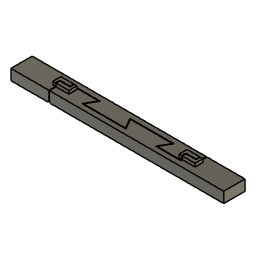
Split Turnout 600mm 15deg (Autodesk Fusion 360 archive; units mm, degrees)
design "Track Joint Parametric"
Autodesk Fusion 360 part; units mm, degrees
sketch "Sketch1" plane through (0, 0, 0) normal (0, 0, 1) x (1, 0, 0)
  line L0 (-20, 2) -> (20, 2)
  line L1 (20, 2) -> (20, -2)
  line L2 (20, -2) -> (-20, -2)
  line L3 (-20, -2) -> (-20, 2)
  line L4 (0, -2) -> (0, 2) construction
  line L5 (-20, 0) -> (20, 0) construction
  line L6 (-11.85, 2) -> (-11.85, -2) construction
  line L7 (11.85, 2) -> (11.85, -2) construction
  line L8 (-12.75, 2) -> (-12.75, -2)
  line L9 (-12.45, 2) -> (-12.45, -2) construction
  line L10 (-11.25, 2) -> (-11.25, -2) construction
  line L11 (-10.95, 2) -> (-10.95, -2)
  line L12 (11.25, 2) -> (11.25, -2) construction
  line L13 (12.45, 2) -> (12.45, -2) construction
  line L14 (10.95, 2) -> (10.95, -2)
  line L15 (12.75, 2) -> (12.75, -2)
  line L16 (-13.35, 0.75) -> (-10.35, 0.75)
  line L17 (-10.35, 0.75) -> (-10.35, -0.75)
  line L18 (-10.35, -0.75) -> (-13.35, -0.75)
  line L19 (-13.35, -0.75) -> (-13.35, 0.75)
  line L20 (10.35, 0.75) -> (13.35, 0.75)
  line L21 (13.35, 0.75) -> (13.35, -0.75)
  line L22 (13.35, -0.75) -> (10.35, -0.75)
  line L23 (10.35, -0.75) -> (10.35, 0.75)
  line L24 (-11.85, 1) -> (-6.3453, 1) construction
  line L25 (-6.3453, 1) -> (-7.5, -1) construction
  line L26 (-7.5, -1) -> (0.5774, -1) construction
  line L27 (0.5774, -1) -> (-0.5774, 1) construction
  line L28 (-0.5774, 1) -> (7.5, 1) construction
  line L29 (7.5, 1) -> (6.3453, -1) construction
  line L30 (6.3453, -1) -> (11.85, -1) construction
  line L31 (-3.4613, -1) -> (-3.4613, 2) construction
  line L32 (3.4613, 1) -> (3.4613, -2) construction
  line L33 (-12.85, 0.05) -> (-10.95, 0.05)
  line L34 (-10.95, 1.05) -> (-6.2587, 1.05)
  line L35 (-6.2587, 1.05) -> (-7.4134, -0.95)
  line L36 (-7.4134, -0.95) -> (0.4907, -0.95)
  line L37 (0.4907, -0.95) -> (-0.664, 1.05)
  line L38 (-0.664, 1.05) -> (7.5866, 1.05)
  line L39 (7.5866, 1.05) -> (6.4319, -0.95)
  line L40 (6.4319, -0.95) -> (10.85, -0.95)
  line L41 (-12.85, 0.05) -> (-12.85, -2)
  line L42 (-12.75, -0.05) -> (-10.85, -0.05)
  line L43 (-10.85, -0.05) -> (-10.85, 0.95)
  line L44 (-10.85, 0.95) -> (-6.4319, 0.95)
  line L45 (-6.4319, 0.95) -> (-7.5866, -1.05)
  line L46 (-7.5866, -1.05) -> (0.664, -1.05)
  line L47 (0.664, -1.05) -> (-0.4907, 0.95)
  line L48 (-0.4907, 0.95) -> (7.4134, 0.95)
  line L49 (7.4134, 0.95) -> (6.2587, -1.05)
  line L50 (6.2587, -1.05) -> (10.95, -1.05)
  line L51 (10.85, -0.95) -> (10.85, -0.903)
  line L52 (10.85, -0.903) -> (10.85, 0.05)
  line L53 (10.85, 0.05) -> (12.75, 0.05)
  line L54 (10.95, -0.05) -> (12.85, -0.05)
  line L55 (12.85, -0.05) -> (12.85, 2)
  line L56 (-12.25, 2) -> (-12.25, -2) construction
  line L57 (-11.45, -2) -> (-11.45, 2) construction
  line L58 (11.45, 2) -> (11.45, -2) construction
  line L59 (12.25, 2) -> (12.25, -2) construction
  point P0 (-6.9226, 0)
  point P1 (6.9226, 0)
  point P2 (-11.85, 0)
  point P3 (11.85, 0)
  dimension "d123" = 40
  dimension "d124" = 1.2
  dimension "d125" = 1.8
  dimension "d127" = 4
  dimension "d128" = 3
  dimension "d129" = 1.5
  dimension "d130" = 30
  dimension "d131" = 2
  dimension "d132" = 15
  dimension "d133" = 0.1
  dimension "d134" = 0.1
  dimension "d136" = 0.1
  dimension "d137" = 0.1
  dimension "d138" = 0.1
  dimension "d139" = 0.1
  dimension "d140" = 0.1
  dimension "d141" = 0.1
  dimension "d142" = 0.1
  dimension "d143" = 0.1
  dimension "d144" = 0.1
  dimension "d145" = 0.1
  dimension "d146" = 0.1
  dimension "d147" = 0.8
  dimension "d161" = 22.5
  constraint horizontal L0
  constraint vertical L1
  constraint horizontal L2
  constraint vertical L3
  constraint coincident L2 L4.start
  constraint coincident L0 L4.end
  constraint coincident L3 L5.start
  constraint coincident L1 L5.end
  constraint perpendicular L0 L4
  constraint perpendicular L1 L5
  constraint symmetric L1 L3 L4
  constraint symmetric L0 L2 L5
  constraint coincident origin L4
  constraint coincident origin L5
  constraint coincident L0 L6.start
  constraint coincident L2 L6.end
  constraint perpendicular L2 L6
  constraint coincident L0 L7.start
  constraint coincident L2 L7.end
  constraint perpendicular L2 L7
  constraint symmetric L4 L6 L7
  constraint coincident L0 L8.start
  constraint coincident L2 L8.end
  constraint perpendicular L2 L8
  constraint coincident L0 L9.start
  constraint coincident L2 L9.end
  constraint perpendicular L2 L9
  constraint coincident L0 L10.start
  constraint coincident L2 L10.end
  constraint perpendicular L2 L10
  constraint coincident L0 L11.start
  constraint coincident L2 L11.end
  constraint perpendicular L2 L11
  constraint symmetric L6 L9 L10
  constraint symmetric L6 L8 L11
  constraint coincident L0 L12.start
  constraint coincident L2 L12.end
  constraint perpendicular L2 L12
  constraint coincident L0 L13.start
  constraint coincident L2 L13.end
  constraint perpendicular L2 L13
  constraint coincident L0 L14.start
  constraint coincident L2 L14.end
  constraint perpendicular L2 L14
  constraint coincident L0 L15.start
  constraint coincident L2 L15.end
  constraint perpendicular L2 L15
  constraint symmetric L7 L14 L15
  constraint symmetric L7 L12 L13
  constraint symmetric L4 L11 L14
  constraint symmetric L4 L10 L12
  constraint horizontal L16
  constraint vertical L17
  constraint horizontal L18
  constraint vertical L19
  constraint symmetric L5 L16 L18
  constraint symmetric L6 L17 L19
  constraint horizontal L20
  constraint vertical L21
  constraint horizontal L22
  constraint vertical L23
  constraint symmetric L5 L20 L22
  constraint symmetric L7 L21 L23
  constraint symmetric L4 L17 L23
  constraint collinear L18 L22
  constraint coincident L6 L24.start
  constraint coincident L7 L30.end
  constraint parallel L5 L30
  constraint parallel L5 L28
  constraint parallel L5 L26
  constraint parallel L5 L24
  constraint coincident origin L27
  constraint collinear L26 L30
  constraint coincident L25 P0
  constraint coincident L29 P1
  constraint coincident L5 P1
  constraint coincident L5 P0
  constraint symmetric L4 P0 P1
  constraint coincident L26 L31.start
  constraint coincident L0 L31.end
  constraint perpendicular L0 L31
  constraint symmetric L25 L27 L31
  constraint coincident L28 L32.start
  constraint coincident L2 L32.end
  constraint perpendicular L2 L32
  constraint symmetric L27 L29 L32
  constraint coincident L11 L33.end
  constraint perpendicular L11 L33
  constraint coincident L11 L34.start
  constraint parallel L30 L40
  constraint parallel L29 L39
  constraint parallel L28 L38
  constraint parallel L27 L37
  constraint parallel L26 L36
  constraint parallel L25 L35
  constraint parallel L24 L34
  constraint coincident L2 L41.end
  constraint parallel L8 L41
  constraint coincident L8 L42.start
  constraint parallel L26 L46
  constraint parallel L25 L45
  constraint parallel L24 L44
  constraint parallel L11 L43
  constraint parallel L33 L42
  constraint parallel L28 L48
  constraint parallel L29 L49
  constraint parallel L30 L50
  constraint parallel L27 L47
  constraint coincident L14 L50.end
  constraint perpendicular L40 L51
  constraint coincident L15 L53.end
  constraint coincident L14 L54.start
  constraint coincident L0 L55.end
  constraint parallel L15 L55
  constraint parallel L5 L54
  constraint parallel L53 L54
  constraint parallel L14 L52
  constraint coincident L0 L56.start
  constraint perpendicular L0 L56
  constraint coincident L2 L56.end
  constraint coincident L2 L57.start
  constraint coincident L0 L57.end
  constraint perpendicular L0 L57
  constraint symmetric L6 L56 L57
  constraint coincident L0 L58.start
  constraint coincident L2 L58.end
  constraint perpendicular L2 L58
  constraint coincident L0 L59.start
  constraint coincident L2 L59.end
  constraint perpendicular L2 L59
  constraint symmetric L7 L58 L59
  constraint symmetric L4 L57 L58
  constraint coincident L6 P2
  constraint coincident L5 P2
  constraint coincident L7 P3
  constraint coincident L5 P3
  measures "d123" distance of L1 L3
  measures "d124" distance of L9 L10
  measures "d125" distance of L8 L11
  measures "d127" distance of L0 L2
  measures "d128" distance of L17 L19
  measures "d129" distance of L16 L18
  measures "d130" angle of L4 L27
  measures "d131" distance of L28 L30
  measures "d132" horizontal distance of L25.end L28.end
  measures "d133" distance of L37 L47
  measures "d134" distance of L38 L48
  measures "d136" distance of L36 L46
  measures "d137" distance of L35 L45
  measures "d138" distance of L39 L49
  measures "d139" distance of L40 L50
  measures "d140" distance of L34 L44
  measures "d141" distance of L11 L43
  measures "d142" distance of L33 L42
  measures "d143" distance of L8 L41
  measures "d144" distance of L53 L54
  measures "d145" distance of L14 L52
  measures "d146" distance of L15 L55
  measures "d147" distance of L56 L57
  measures "d161" distance of L10 L12
sketch "Sketch2" plane through (0, 0, 0) normal (0, 1, 0) x (1, 0, 0)
  line L0 (10.95, 0) -> (12.75, 0)
  line L1 (12.75, 0) -> (12.75, -0.3)
  line L2 (12.75, -0.3) -> (12.25, -0.3)
  line L3 (12.25, -0.3) -> (12.25, -1.8)
  line L4 (12.25, -1.8) -> (12.45, -1.8)
  line L5 (12.45, -1.8) -> (12.45, -2.4)
  line L6 (12.45, -2.4) -> (11.25, -2.4)
  line L7 (11.25, -2.4) -> (11.25, -1.8)
  line L8 (11.25, -1.8) -> (11.45, -1.8)
  line L9 (11.45, -1.8) -> (11.45, -0.3)
  line L10 (11.45, -0.3) -> (10.95, -0.3)
  line L11 (10.95, -0.3) -> (10.95, 0)
  line L12 (11.85, 0) -> (11.85, -2.4) construction
  line L13 (-12.45, -1.8) -> (-12.25, -1.8)
  line L14 (-10.95, 0) -> (-10.95, -0.3)
  line L15 (-11.45, -0.3) -> (-11.45, -1.8)
  line L16 (-12.25, -1.8) -> (-12.25, -0.3)
  line L17 (-10.95, -0.3) -> (-11.45, -0.3)
  line L18 (-12.75, -0.3) -> (-12.75, 0)
  line L19 (-12.75, 0) -> (-10.95, 0)
  line L20 (-11.25, -1.8) -> (-11.25, -2.4)
  line L21 (-11.85, 0) -> (-11.85, -2.4) construction
  line L22 (-12.25, -0.3) -> (-12.75, -0.3)
  line L23 (-12.45, -2.4) -> (-12.45, -1.8)
  line L24 (-11.45, -1.8) -> (-11.25, -1.8)
  line L25 (-11.25, -2.4) -> (-12.45, -2.4)
  point P0 (11.85, 0)
  point P1 (12.45, 0)
  point P2 (12.75, 0)
  point P3 (12.25, 0)
  point P4 (-11.85, 0)
  point P5 (-11.45, 0)
  point P6 (-11.25, 0)
  point P7 (-10.95, 0)
  dimension "d148" = 2.4
  dimension "d149" = 1.2
  dimension "d150" = 0.6
  dimension "d151" = 0.3
  constraint horizontal L0
  constraint perpendicular L0 L1
  constraint perpendicular L1 L2
  constraint perpendicular L2 L3
  constraint perpendicular L1 L4
  constraint perpendicular L2 L5
  constraint perpendicular L5 L6
  constraint perpendicular L6 L7
  constraint perpendicular L7 L8
  constraint perpendicular L8 L9
  constraint perpendicular L9 L10
  constraint perpendicular L10 L11
  constraint coincident L0 P0
  constraint coincident L6 L12.end
  constraint perpendicular L6 L12
  constraint symmetric L1 L11 L12
  constraint symmetric L3 L9 L12
  constraint collinear L4 L8
  constraint collinear L2 L10
  constraint coincident P0 L12.start
  constraint coincident L0.end L1.start
  constraint symmetric L5 L7 L12
  constraint coincident L3 P3
  constraint coincident L5 P1
  constraint horizontal L19
  constraint perpendicular L14 L19
  constraint perpendicular L14 L17
  constraint perpendicular L15 L17
  constraint perpendicular L14 L24
  constraint perpendicular L17 L20
  constraint perpendicular L20 L25
  constraint perpendicular L23 L25
  constraint perpendicular L13 L23
  constraint perpendicular L13 L16
  constraint perpendicular L16 L22
  constraint perpendicular L18 L22
  constraint coincident L21.end L25
  constraint perpendicular L21 L25
  constraint symmetric L14 L18 L21
  constraint symmetric L15 L16 L21
  constraint collinear L13 L24
  constraint collinear L17 L22
  constraint symmetric L20 L21 L23
  constraint coincident L15 P5
  constraint coincident L20 P6
  constraint coincident P4 L19
  constraint coincident P4 L21.start
  constraint coincident P7 L14.start
  constraint collinear L10 L17
  constraint collinear L8 L24
  constraint collinear L6 L25
  measures "d148" distance of L0 L6
  measures "d149" distance of L5 L7
  measures "d150" distance of L4 L6
  measures "d151" distance of L0 L2
extrude "Extrude2" add sketch "Sketch1" against normal blind 2 contours L0 L2 L3 L8 L16 L18 L19 L41 | L0 L8 L11 L16 | L0 L11 L14 L20 L22 L23 L34 L35 L36 L37 L38 L39 L40 L51 L52 | L8 L11 L16 L33 | L8 L16 L18 L19 L33 L41 | L0 L14 L15 L20 | L14 L15 L20 L53 | L14 L20 L22 L23 L52 L53 makes body 1
extrude "Extrude3" add sketch "Sketch1" along normal blind 0.6 contours L8 L11 L16 L33 | L8 L16 L18 L19 L33 L41 | L14 L15 L20 L53 | L14 L20 L22 L23 L52 L53 bodies 1
extrude "Extrude1" add sketch "Sketch1" against normal up to surface (2 mm away) separate body contours L2 L8 L11 L18 | L8 L11 L18 L42 | L2 L11 L14 L16 L17 L18 L43 L44 L45 L46 L47 L48 L49 L50 | L11 L16 L17 L18 L42 L43 | L0 L1 L2 L15 L20 L21 L22 L55 | L2 L14 L15 L22 | L15 L20 L21 L22 L54 L55 | L14 L15 L22 L54 makes body 2 in component "Join 2"
extrude "Extrude2'" add sketch "Sketch1" along normal up to surface (0.6 mm away) contours L8 L11 L18 L42 | L11 L16 L17 L18 L42 L43 | L15 L20 L21 L22 L54 L55 | L14 L15 L22 L54 bodies 2 in component "Join 2"
chamfer "Chamfer2" distance 0.2 angle 45 13 edges at (-12.85, -0.975, -2) (-11.9, 0.05, -2) (-10.95, 0.55, -2) (-8.6043, 1.05, -2) (-6.836, 0.05, -2) (-3.4613, -0.95, -2) (-0.0866, 0.05, -2) (3.4613, 1.05, -2) (7.0093, 0.05, -2) (8.641, -0.95, -2) (10.85, -0.45, -2) (11.8, 0.05, -2) (12.75, 1.025, -2) measured on face at (-17.6167, 0.0167, -2) measured on face at (-17.6167, 0.0167, -2) measured on face at (-17.6167, 0.0167, -2) measured on face at (-17.6167, 0.0167, -2) measured on face at (-17.6167, 0.0167, -2) measured on face at (-17.6167, 0.0167, -2) measured on face at (-17.6167, 0.0167, -2) measured on face at (-17.6167, 0.0167, -2) measured on face at (-17.6167, 0.0167, -2) measured on face at (-17.6167, 0.0167, -2) measured on face at (-17.6167, 0.0167, -2) measured on face at (-17.6167, 0.0167, -2) measured on face at (-17.6167, 0.0167, -2) on bodies 1
chamfer "Chamfer1" distance 0.2 angle 45 13 edges at (-12.75, -1.025, -2) (-11.8, -0.05, -2) (-10.85, 0.45, -2) (-8.641, 0.95, -2) (-7.0093, -0.05, -2) (-3.4613, -1.05, -2) (0.0866, -0.05, -2) (3.4613, 0.95, -2) (6.836, -0.05, -2) (8.6043, -1.05, -2) (10.95, -0.55, -2) (11.9, -0.05, -2) (12.85, 0.975, -2) measured on face at (-12.75, -0.9333, -1.3333) measured on face at (-12.1167, -0.05, -0.2667) measured on face at (-10.85, 0.55, -1.3333) measured on face at (-9.3773, 0.95, -0.6667) measured on face at (-6.8168, 0.2833, -0.6667) measured on face at (-4.8364, -1.05, -0.6667) measured on face at (0.2791, -0.3833, -0.6667) measured on face at (2.144, 0.95, -0.6667) measured on face at (6.6436, -0.3833, -1.3333) measured on face at (7.8225, -1.05, -0.6667) measured on face at (10.95, -0.6167, -1.3333) measured on face at (11.5833, -0.05, -0.2667) measured on face at (12.85, 0.9, -1.3333) on bodies 2 in component "Join 2"
component "Join 2" placed x (1, 0, 0) y (0, 1, 0) z (0, 0, 1) at (0, 0, 0)
equation "Gauge = 22.5 mm"
equation "SleeperThickness = 2 mm"
equation "Tollerance = 0.1 mm"
equation "d105 = -SleeperThickness"
equation "SleeperSpcing = Gauge / 1.5"
equation "d115 = Gauge / 37.5"
equation "d123 = d127 * 10"
equation "d124 = Gauge / 18.75"
equation "d125 = d124 * 1.5"
equation "d126 = Gauge"
equation "d127 = Gauge / 5.625"
equation "d128 = d124 * 2.5"
equation "d129 = d128 / 2"
equation "d130 = 30 °"
equation "d131 = d127 / 2"
equation "d132 = d161 / 1.5"
equation "d133 = Tollerance"
equation "d134 = d133"
equation "d136 = d133"
equation "d137 = d133"
equation "d138 = d133"
equation "d139 = d133"
equation "d140 = d133"
equation "d141 = d133"
equation "d142 = d133"
equation "d143 = d133"
equation "d144 = d133"
equation "d145 = d133"
equation "d146 = d133"
equation "d147 = d124 / 1.5"
equation "d148 = d149 * 2"
equation "d150 = d149 / 2"
equation "d151 = d149 / 4"
equation "d160 = Gauge"
equation "d161 = Gauge"
named bodies: "Joint 1"
